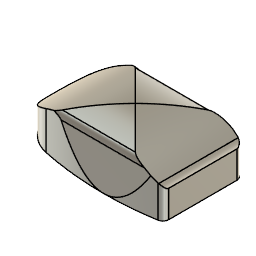
24 (Autodesk Fusion 360 design; units mm, degrees)
Autodesk Fusion 360 part; units mm, degrees
sketch "草图1" plane through (0, 0, 0) normal (0, 1, 0) x (1, 0, 0)
  line L0 (0, -55) -> (0, 50) construction
  line L1 (-125, 0) -> (125, 0) construction
  line L2 (-31, 0) -> (20, 0)
  circle A0 centre (20, -1) radius 1
  arc A1 (-31.065, -5.889) -> (18.5199, -10.8983) centre (-3, 24) ccw
  line L3 (-31.6884, -4.6053) -> (-31.9962, -1.0872)
  line L4 (20.4052, -7.8422) -> (20.9962, -1.0872)
  line L5 (21, 0) -> (21, -0.6) construction
  line L6 (-32, 0) -> (-32, -0.7) construction
  line L7 (0, -17) -> (10, -17) construction
  arc A2 (-31, 0) -> (-31.9962, -1.0872) centre (-31, -1) ccw
  arc A3 (-31.6884, -4.6053) -> (-31.065, -5.889) centre (-29.696, -4.431) ccw
  arc A4 (-8, 0) -> (8, 0) centre (0, 0) ccw
  arc A5 (18.5199, -10.8983) -> (20.4052, -7.8422) centre (16.4204, -7.4936) ccw
  line L8 (0, -8) -> (0, 0)
  dimension "d1" = 16
  dimension "d2" = 2
  dimension "d3" = 2
  dimension "d4" = 5
  dimension "d5" = 5
  dimension "d6" = 8
  dimension "d7" = 4
  dimension "d8" = 21
  dimension "d9" = 53
  dimension "d10" = 41
  dimension "d11" = 17
  dimension "d12" = 24
  dimension "d13" = 24
  constraint coincident A4.centre L8.end
  constraint vertical L0
  constraint horizontal L1
  constraint coincident L1 L2.start
  constraint coincident L1 L2.end
  constraint tangent L1 A2
  constraint coincident L2.end A0
  constraint tangent L1 A0
  constraint tangent L3 A2
  constraint coincident A0 L4.end
  constraint tangent A0 L4
  constraint tangent L4 A5
  constraint tangent L3 A3
  constraint coincident L1 L5.start
  constraint perpendicular L1 L5
  constraint tangent A0 L5
  constraint coincident L1 L6.start
  constraint perpendicular L1 L6
  constraint tangent L6 A2
  constraint tangent A1 A5
  constraint tangent A1 A3
  constraint horizontal L7
  constraint tangent A1 L7
  constraint coincident L1 A4.end
  constraint coincident L1 A4.start
  constraint midpoint A4 L8.start
  measures "d1" diameter of A4
  measures "d2" diameter of A0
  measures "d3" diameter of A2
  measures "d4" angle of L0 L3
  measures "d5" angle of L0 L4
  measures "d6" diameter of A5
  measures "d7" diameter of A3
  measures "d8" distance of A4.centre L5.start
  measures "d9" distance of L5.start L6.start
  measures "d10" radius of A1
  measures "d11" distance of L2 L7
  measures "d12" distance of L2 A1.centre
  measures "d13" horizontal distance of A1.centre L5.start
extrude "拉伸1" add sketch "草图1" along normal mid plane 30
revolve "旋转1" cut sketch "草图1" angle 360 about axis through (0, 0, 55) along (0, 0, -1) contours L2 A4 L8 picked at (-0.3795, -5.3062)
sketch "草图2" plane through (0, 0, 0) normal (0, 0, 1) x (1, 0, 0)
  line L0 (-31, -15) -> (20, -15)
  line L1 (20, 15) -> (-31, 15)
  arc A0 (18.3234, 13.6051) -> (-20.6815, 12.7204) centre (1.1833, -91) ccw
  arc A1 (-20.6815, -12.7204) -> (18.3234, -13.6051) centre (1.1833, 91) ccw
  line L2 (20, 11.6314) -> (20, -11.6314)
  arc A2 (20, 11.6314) -> (18.3234, 13.6051) centre (18, 11.6314) ccw
  arc A3 (18.3234, -13.6051) -> (20, -11.6314) centre (18, -11.6314) ccw
  arc A4 (-20.6815, 12.7204) -> (-20.6815, -12.7204) centre (-18, 0) ccw
  line L3 (-31, 15) -> (-31, -15) construction
  line L4 (-40, 0) -> (31, 0) construction
  dimension "d17" = 2
  dimension "d18" = 2
  dimension "d19" = 13
  dimension "d20" = 106
  dimension "d21" = 106
  constraint tangent L2 A3
  constraint tangent L2 A2
  constraint tangent A0 A2
  constraint tangent A0 A4
  constraint tangent A1 A4
  constraint tangent A1 A3
  constraint collinear L0.end L1.start L2.start
  constraint collinear L0.end L1.start L2.end
  constraint tangent L1 A0
  constraint tangent L0 A1
  constraint coincident L1.end L3.start
  constraint coincident L0.start L3.end
  constraint tangent A4 L3
  constraint parallel L1 L4
  constraint symmetric A0 A1 L4
  measures "d17" radius of A3
  measures "d18" radius of A2
  measures "d19" radius of A4
  measures "d20" radius of A1
  measures "d21" radius of A0
extrude "拉伸2" cut sketch "草图2" along normal blind 35 keep common part
sketch "草图3" plane through (0, 0, 0) normal (1, 0, 0) x (0, 1, 0)
  line L0 (-15, 0) -> (15, 0)
  line L1 (15, 0) -> (13.8335, 13.3333)
  line L2 (-15, 0) -> (-13.8335, 13.3333)
  line L3 (0, 45) -> (0, -20) construction
  line L4 (-40, 0) -> (40, 0) construction
  arc A0 (12.4483, 15.0645) -> (-12.4483, 15.0645) centre (0, -24) ccw
  arc A1 (-12.4483, 15.0645) -> (-13.8335, 13.3333) centre (-11.8411, 13.159) ccw
  arc A2 (13.8335, 13.3333) -> (12.4483, 15.0645) centre (11.8411, 13.159) ccw
  line L5 (0, 17) -> (10, 17) construction
  dimension "d24" = 10
  dimension "d25" = 30
  dimension "d26" = 4
  dimension "d27" = 4
  dimension "d28" = 41
  dimension "d29" = 17
  constraint horizontal L0
  constraint vertical L3
  constraint horizontal L4
  constraint tangent L1 A2
  constraint tangent A0 A2
  constraint tangent A0 A1
  constraint tangent L2 A1
  constraint symmetric L1 L2 L3
  constraint symmetric L3 A1 A2
  constraint coincident L3 L5.start
  constraint perpendicular L3 L5
  constraint tangent A0 L5
  constraint collinear L0 L4
  measures "d24" angle of L1 L2
  measures "d25" distance of L0.start L0.end
  measures "d26" diameter of A2
  measures "d27" diameter of A1
  measures "d28" radius of A0
  measures "d29" distance of L4 L5
extrude "拉伸3" cut sketch "草图3" along normal mid plane 100 keep common part
